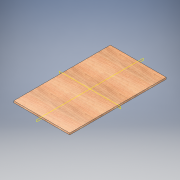
# Autodesk Inventor part: plywoodBase
Saved by Autodesk Inventor 2018.2 (Build 222227000, 227)
## iProperties
Created: 2018-01-07
Part Number: plywoodBase
Material: Wood (Birch)
Document SubType Name: Modeling
Designer: steele
Density: 0.55 g/cm^3
Appearance: Birch - Natural Polished
Mass: 2054.83 g
Surface Area: 6169.41 cm^2
Volume: 3736.05 cm^3
Author: steele
Autodesk Inventor part; units mm, degrees
ref_plane "XZ Plane" through (0, 0, 0) normal (0, 1, 0) x (-1, 0, 0)
sketch "Sketch1" plane through (0, 0, 0) normal (0, 1, 0) x (-1, 0, 0)
  line L0 (206.375, 356.362) -> (-206.375, 356.362)
  line L1 (-206.375, 356.362) -> (-206.375, -356.362)
  line L2 (-206.375, -356.362) -> (206.375, -356.362)
  line L3 (206.375, -356.362) -> (206.375, 356.362)
  line L4 (206.375, 356.362) -> (-206.375, -356.362) construction
  line L5 (-206.375, 356.362) -> (206.375, -356.362) construction
  point P0 (0, 0)
  dimension "d0" = 412.75
  dimension "d1" = 712.724
  constraints: 12 end point, 2 midpoint, 2 parallel, 1 horizontal, 1 perpendicular
  measures "d0" distance of L0.start L0.end
  measures "d1" distance of L1.end L0.end
extrude "Extrusion1" add sketch "Sketch1" along normal blind 12.7
body "Solid1"
